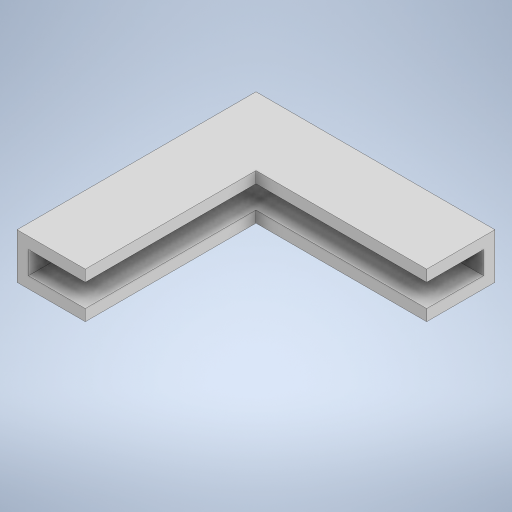
# Autodesk Inventor part: TSU_Corner_Clamp
Saved by Autodesk Inventor 2024 (Build 280153000, 153)
## iProperties
Created: 2025-01-02
Part Number: TSU_Corner_Clamp
Material: Generic
Document SubType Name: Modeling
Designer: Matt Tidd
Density: 1 g/cm^3
Appearance: Default
Author: Matt Tidd
Autodesk Inventor part; units mm, degrees
ref_plane "YZ Plane" through (0, 0, 0) normal (1, 0, 0) x (0, 1, 0)
ref_plane "XZ Plane" through (0, 0, 0) normal (0, 1, 0) x (-1, 0, 0)
ref_plane "XY Plane" through (0, 0, 0) normal (0, 0, 1) x (1, 0, 0)
sketch "Sketch2" plane through (0, 0, 0) normal (0, 1, 0) x (-1, 0, 0)
  line L0 (0, 0) -> (0, 75)
  line L1 (0, 75) -> (30, 75)
  line L2 (30, 75) -> (30, 0)
  line L3 (0, 0) -> (-75, 0)
  line L4 (0, 0) -> (75, 0) construction
  line L5 (-75, 0) -> (-75, -30)
  line L6 (-75, -30) -> (30, -30)
  line L7 (30, -30) -> (30, 0)
  dimension "d7" = 75
  dimension "d8" = 30
  dimension "d9" = 90
  dimension "d10" = 75
  dimension "d11" = 90
  dimension "d12" = 75
  dimension "d13" = 180
  dimension "d14" = 30
  dimension "d15" = 90
  constraints: 16 end point, 4 perpendicular, 2 collinear, 2 horizontal, 1 vertical
  measures "d7" distance of L0.start L0.end
  measures "d8" distance of L0.end L1.end
  measures "d9" angle of L0 L1
  measures "d10" distance of L1.end L2.end
  measures "d11" angle of L1 L2
  measures "d12" distance of L0.start L3.end
  measures "d13" angle of L3 L4
  measures "d14" distance of L3.end L5.end
  measures "d15" angle of L5 L3
extrude "Extrusion1" add sketch "Sketch2" along normal blind 20
sketch "Sketch3" plane through (0, 0, 75) normal (1, 0, 0) x (0, 0, -1)
  line L0 (0, 5) -> (75, 5)
  line L1 (75, 5) -> (75, 15)
  line L2 (75, 15) -> (0, 15)
  line L3 (0, 15) -> (0, 5)
  point P0 (75, 0)
  dimension "d18" = 10
  constraints: 8 end point, 2 parallel, 1 horizontal, 1 perpendicular
  measures "d18" distance of L1.end L0.end
extrude "Extrusion2" cut sketch "Sketch3" against normal blind 25
sketch "Sketch4" plane through (0, 0, 0) normal (0, 0, 1) x (1, 0, 0)
  line L0 (0, 15) -> (-25, 15) projected
  line L1 (-25, 15) -> (75, 15)
  line L2 (75, 15) -> (75, 5)
  line L3 (75, 5) -> (-25, 5)
  line L4 (-25, 5) -> (-25, 15)
  point P0 (0, 0)
  dimension "d21" = 100
  dimension "d22" = 10
  constraints: 8 end point, 2 parallel, 1 horizontal, 1 perpendicular
  measures "d21" distance of L2.end L3.end
  measures "d22" distance of L1.end L2.end
extrude "Extrusion3" cut sketch "Sketch4" against normal blind 25
body "Solid1"
